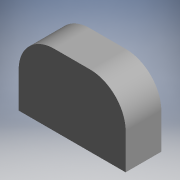
# Autodesk Inventor part: arc_test
Saved by Autodesk Inventor 2019 (Build 230136000, 136)
## iProperties
Part Number: arc_test
Material: Generic
Document SubType Name: Modeling
Designer: oriani
Appearance: Default
Author: oriani
Autodesk Inventor part; units mm, degrees
ref_plane "YZ Plane" through (0, 0, 0) normal (1, 0, 0) x (0, 1, 0)
ref_plane "XZ Plane" through (0, 0, 0) normal (0, 1, 0) x (-1, 0, 0)
ref_plane "XY Plane" through (0, 0, 0) normal (0, 0, 1) x (1, 0, 0)
sketch "Sketch1" plane through (0, 0, 0) normal (0, 0, 1) x (1, 0, 0)
  line L0 (0, 0) -> (0, 25.4)
  arc A0 (0, 25.4) -> (-25.4, 50.8) centre (-25.4, 25.4) ccw
  line L1 (-25.4, 50.8) -> (-50.8, 50.8)
  arc A1 (-50.8, 50.8) -> (-76.2, 25.4) centre (-50.8, 25.4) ccw
  line L2 (-76.2, 25.4) -> (-76.2, 0)
  line L3 (-76.2, 0) -> (0, 0)
  point P0 (-38.1, 12.7)
  constraints: 8 end point, 4 point on circle, 2 centre point
extrude "Extrusion1" add sketch "Sketch1" along normal blind 25.4
hole "Hole1" at (-38.1, 12.7, 0) direction (0, 0, 1) diameter 3.9624 depth 12.7 tip angle 118 thread size "10-32 UNF" class "2B" standard "ANSI Unified Screw Threads"
body "Solid1"
